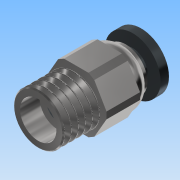
# Autodesk Inventor part: фитинг
Saved by Autodesk Inventor 2017 (Build 210142000, 142)
## iProperties
Part Number: фитинг
Material: Типовые
Document SubType Name: Modeling
Designer: Max
Mass: 0.908248 g
Surface Area: 15.3164 cm^2
Volume: 0.908248 cm^3
Density: 1 g/cm^3
Appearance: Сталь — полированная
Author: Max
Autodesk Inventor part; units mm, degrees
ref_plane "YZ Plane" through (0, 0, 0) normal (1, 0, 0) x (0, 1, 0)
ref_plane "XZ Plane" through (0, 0, 0) normal (0, 1, 0) x (-1, 0, 0)
ref_plane "XY Plane" through (0, 0, 0) normal (0, 0, 1) x (1, 0, 0)
sketch "Эскиз1" plane through (0, 0, 0) normal (0, 0, 1) x (1, 0, 0)
  line L0 (0, 0) -> (0, 141.677) construction
  line L1 (0, 0) -> (-115.9774, 0) construction
  line L2 (-3.25, 0) -> (-3.25, 3.5)
  line L3 (-3.25, 3.5) -> (-2, 3.5)
  line L4 (-2, 3.5) -> (-2, 18.75)
  line L5 (-5, 18.4) -> (-5, 16.9)
  line L6 (-5, 16.9) -> (-2.7, 16.9)
  line L7 (-2.7, 16.9) -> (-2.7, 15.7)
  line L8 (-2.7, 15.7) -> (-3.85, 15.7)
  line L9 (-3.85, 15.7) -> (-3.85, 15)
  line L10 (-5, 13) -> (-5, 6.8)
  line L11 (-5, 6.8) -> (-4.5, 6.8)
  line L12 (-4.5, 6.8) -> (-4.5, 0)
  line L13 (-3.25, 0) -> (-4.5, 0)
  arc A0 (-4.0555, 15) -> (-5, 13) centre (-2.4102, 13) ccw
  line L14 (-4.0555, 15) -> (-3.85, 15)
  arc A1 (-2, 18.75) -> (-5, 18.4) centre (-2, 5.7179) ccw
  line L15 (-2, 18.75) -> (0, 18.75) construction
  dimension "d0" = 3.25
  dimension "d1" = 4.5
  dimension "d2" = 5
  dimension "d3" = 6.8
  dimension "d4" = 3.5
  dimension "d5" = 6.2
  dimension "d6" = 3.85
  dimension "d7" = 2
  dimension "d8" = 0.7
  dimension "d9" = 1.2
  dimension "d10" = 2.7
  dimension "d11" = 1.5
  dimension "d12" = 2
  dimension "d13" = 18.75
  dimension "d14" = 15.7
  dimension "d15" = 2.7
  dimension "d16" = 13
  dimension "d17" = 5
  constraints: 32 end point, 9 perpendicular, 4 point on circle, 4 point on line, 3 vertical, 2 centre point, 2 horizontal, 2 tangent
  measures "d0" distance between parallel lines of L0 L2
  measures "d1" distance between parallel lines of L0 L12
  measures "d2" distance between parallel lines of L0 L10
  measures "d3" distance between parallel lines of L13 L11
  measures "d4" distance between parallel lines of L1 L3
  measures "d5" distance of L10.start L10.end
  measures "d6" distance between parallel lines of L0 L9
  measures "d7" vertical distance of L10.start L9.end
  measures "d8" distance between parallel lines of L14 L8
  measures "d9" distance between parallel lines of L8 L6
  measures "d10" distance between parallel lines of L0 L7
  measures "d11" distance from line of L6 L5.start
  measures "d12" distance between parallel lines of L0 L4
  measures "d13" distance between parallel lines of L1 L15
  measures "d14" distance between parallel lines of L1 L8
  measures "d15" distance from line of L10.start L8
  measures "d16" distance from line of L1 L10.start
  measures "d17" distance between parallel lines of L0 L5
revolve "Вращение1" add sketch "Эскиз1" angle 360 about axis through (0, 0, 0) along (0, 1, 0)
chamfer "Фаска1" distance 0.2 angle 45 1 edges at (4.5, 0, 0)
sketch "Эскиз2" plane through (0, 6.8, 0) normal (0, -1, 0) x (1, 0, 0)
  line L0 (5.7735, 0) -> (2.8868, -5)
  line L1 (2.8868, -5) -> (-2.8868, -5)
  line L2 (-2.8868, -5) -> (-5.7735, 0)
  line L3 (-5.7735, 0) -> (-2.8868, 5)
  line L4 (-2.8868, 5) -> (2.8868, 5)
  line L5 (2.8868, 5) -> (5.7735, 0)
  circle A0 centre (0, 0) radius 4.3
  circle A1 centre (0, 0) radius 5 projected
  dimension "d22" = 10
  constraints: 12 end point, 2 coincident, 1 centre point, 13 other
  measures "d22" distance between parallel lines of L3 L0
extrude "Выдавливание1" add sketch "Эскиз2" against normal blind 6
chamfer "Фаска2" distance 0.7 angle 45 6 edges at (2.8868, 9.8, 5) (5.7735, 9.8, 0) (-2.8868, 9.8, 5) (2.8868, 9.8, -5) (-5.7735, 9.8, 0) (-2.8868, 9.8, -5)
thread "Резьба1" size "M9x1.25" class "6g" standard "ANSI Metric M Profile" full length
sketch "Эскиз4" plane through (0, 6.8, 0) normal (1, 0, 0) x (0, 0, 1)
  line L0 (4.5, 0) -> (4.5, 6.6)
  line L1 (4.5, 6.6) -> (3.5732, 6.6)
  line L2 (3.5732, 6.6) -> (3.5732, 0)
  line L3 (3.5732, 0) -> (4.5, 0)
  line L4 (0, -15.7) -> (0, 10.55) projected
  constraints: 8 end point
revolve "Вращение2" cut sketch "Эскиз4" angle 360 about axis through (0, 6.8, 0) along (0, -1, 0)
sketch "Эскиз5" plane through (0, 6.8, 0) normal (1, 0, 0) x (0, 0, 1)
  line L0 (4.5, 0) -> (4.5, 6.6)
  line L1 (4.5, 6.6) -> (3.5732, 6.6)
  line L2 (3.5732, 6.6) -> (3.5732, 0)
  line L3 (3.5732, 0) -> (4.5, 0)
  line L4 (0, -15.7) -> (0, 10.55) projected
  constraints: 8 end point
revolve "Вращение3" add sketch "Эскиз5" angle 360 about axis through (0, 6.8, 0) along (0, -1, 0) separate body
sketch "Эскиз3" plane through (0, 6.8, 0) normal (-1, 0, 0) x (0, -1, 0)
  line L0 (-0.7293, -3.6366) -> (-0.6251, -3.6366) construction
  line L1 (0.1041, -4.437) -> (-0.0001, -4.6371) construction
  line L2 (-1.2501, -4.6371) -> (-1.3543, -4.437) construction
  line L3 (-0.5209, -3.6366) -> (-0.6251, -3.4364) construction
  line L4 (-0.6251, -3.4364) -> (-0.7293, -3.6366) construction
  line L5 (-1.2501, -4.6371) -> (-1.1459, -4.437) construction
  line L6 (-0.5209, -3.6366) -> (-0.1043, -4.437)
  line L7 (-1.3543, -4.437) -> (-1.1459, -4.437) construction
  arc A0 (-1.3543, -4.437) -> (-1.2501, -4.5002) centre (-1.2501, -4.3827) ccw construction
  line L8 (0.1041, -4.437) -> (-0.1043, -4.437) construction
  line L9 (-1.2501, -4.6371) -> (-1.2501, -4.437) construction
  line L10 (-0.0001, -4.6371) -> (-0.0001, -4.437) construction
  line L11 (-0.6251, -3.4364) -> (-0.6251, -3.5733) construction
  line L12 (-1.2501, -4.5002) -> (-0.0001, -4.5002)
  arc A1 (-1.2501, -4.5002) -> (-1.1459, -4.437) centre (-1.2501, -4.3827) ccw
  line L13 (-0.1043, -4.437) -> (-0.0001, -4.6371) construction
  line L14 (-1.1459, -4.437) -> (-0.7293, -3.6366)
  line L15 (-0.0001, -0.0002) -> (-0.0001, 0.0177)
  line L16 (-0.0001, 0.0177) -> (-0.0001, -0.0002)
  line L17 (-0.0001, -0.0002) -> (0.0334, -0.0002)
  arc A2 (-0.1043, -4.437) -> (-0.0001, -4.5002) centre (-0.0001, -4.3827) ccw
  arc A3 (-0.0001, -4.5002) -> (0.1041, -4.437) centre (-0.0001, -4.3827) ccw construction
  arc A4 (-0.6251, -3.5733) -> (-0.7293, -3.6366) centre (-0.6251, -3.6908) ccw
  arc A5 (-0.5209, -3.6366) -> (-0.6251, -3.5733) centre (-0.6251, -3.6908) ccw
  line L18 (-0.6251, -3.5733) -> (-0.6251, -3.6366) construction
  line L19 (-0.6251, -3.6366) -> (-0.5209, -3.6366) construction
  dimension "d30" = 55
  dimension "d31" = 0.2001
  dimension "d32" = 0.2001
  dimension "Эскиз3_ThreadOffset" = 0
  dimension "Эскиз3_MajorRadius" = 4.5
  dimension "d35" = 1.25
  dimension "Эскиз3_MinorRadius" = 3.5732
  constraints: 40 end point, 12 point on circle, 10 parallel, 8 tangent, 6 centre point, 6 collinear, 2 midpoint, 2 point on line, 1 horizontal, 1 perpendicular, 3 other
  measures "d30" angle of L6 L14
  measures "d31" distance of L3.end L0.end
  measures "d32" distance of L1.end L10.end
  measures "Эскиз3_ThreadOffset" distance between parallel lines of L15 L10
  measures "Эскиз3_MajorRadius" distance from line of L12 L15.start
  measures "d35" distance from line of L1.end L9
  measures "Эскиз3_MinorRadius" distance edge to line of A5 L17
coil "Пружина1" sketch "Эскиз3" operation cut axis through (0, 6.8, 0) along (0, -1, 0) pitch 1.2513 turns 7.272727 hand right bodies 2
equation "\"d30\" = d37"
equation "\"d31\" = 0.160083 * Эскиз3_Pitch"
equation "\"d32\" = 0.160083 * Эскиз3_Pitch"
equation "\"d35\" = Эскиз3_Pitch"
equation "\"d37\" = 55deg"
equation "\"Эскиз3_Pitch\" = 1.25"
